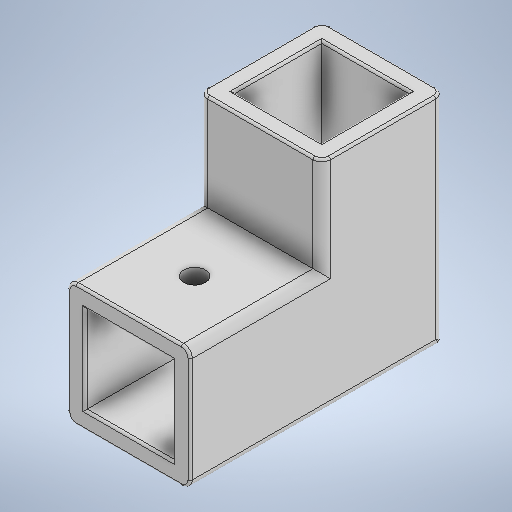
# Autodesk Inventor part: fixed_joint
Saved by Autodesk Inventor 2025 (Build 290162000, 162)
## iProperties
Created: 2024-07-12
Part Number: fixed_joint
Material: Generic
Document SubType Name: Modeling
Designer: hifzhil
Density: 1 g/cm^3
Appearance: Default
Author: hifzhil
Autodesk Inventor part; units mm, degrees
sketch "Sketch1" plane through (0, 0, 0) normal (0, 0, 1) x (1, 0, 0)
  line L0 (-11.6216, -5.5135) -> (8.3784, -5.5135)
  line L1 (8.3784, -5.5135) -> (8.3784, -25.5135)
  line L2 (8.3784, -25.5135) -> (-11.6216, -25.5135)
  line L3 (-11.6216, -25.5135) -> (-11.6216, -5.5135)
  line L4 (-15.6216, -1.5135) -> (12.3784, -1.5135)
  line L5 (12.3784, -1.5135) -> (12.3784, -29.5135)
  line L6 (12.3784, -29.5135) -> (-15.6216, -29.5135)
  line L7 (-15.6216, -29.5135) -> (-15.6216, -1.5135)
  point P0 (0, 0)
  dimension "d0" = 20
  dimension "d1" = 20
  dimension "d2" = 4
  dimension "d3" = 4
  dimension "d4" = 4
  dimension "d5" = 4
  constraints: 16 end point, 4 parallel, 2 horizontal, 2 perpendicular
  measures "d0" distance of L0.end L1.end
  measures "d1" distance of L0.start L0.end
  measures "d2" distance between parallel lines of L0 L4
  measures "d3" distance between parallel lines of L6 L2
  measures "d4" distance between parallel lines of L7 L3
  measures "d5" distance between parallel lines of L5 L1
extrude "Extrusion1" add sketch "Sketch1" along normal blind 30
ref_plane "Work Plane3" through (-15.6216, -29.5135, 0) normal (0, -1, 0) x (1, 0, 0)
sketch "Sketch2" plane through (-15.6216, -29.5135, 0) normal (0, -1, 0) x (1, 0, 0)
  line L0 (0, 0) -> (28, 0)
  line L1 (28, 0) -> (28, -28)
  line L2 (28, -28) -> (0, -28)
  line L3 (0, -28) -> (0, 0)
  line L4 (24, -24) -> (4, -24)
  line L5 (4, -24) -> (4, -4)
  line L6 (4, -4) -> (24, -4)
  line L7 (24, -4) -> (24, -24)
  point P0 (15.6216, 0)
  point P1 (0, -14)
  dimension "d10" = 28
  dimension "d11" = 28
  dimension "d12" = 4
  dimension "d13" = 4
  dimension "d14" = 4
  dimension "d15" = 4
  constraints: 16 end point, 4 parallel, 2 horizontal, 2 perpendicular, 1 midpoint
  measures "d10" distance of L0.end L1.end
  measures "d11" distance of L1.end L2.end
  measures "d12" distance between parallel lines of L1 L7
  measures "d13" distance from line of point (0, -14) L5
  measures "d14" distance between parallel lines of L4 L2
  measures "d15" distance between parallel lines of L0 L6
extrude "Extrusion2" add sketch "Sketch2" against normal blind 50
ref_plane "Work Plane4" through (12.3784, -29.5135, -28) normal (0, 0, -1) x (-1, 0, 0)
sketch "Sketch3" plane through (12.3784, -29.5135, -28) normal (0, 0, -1) x (-1, 0, 0)
  circle A0 centre (14, 35) radius 2.5
  circle A1 centre (14, 15) radius 2.5
  line L0 (28, 0) -> (28, 50) projected
  line L1 (28, 0) -> (0, 0) projected
  point P0 (12.3784, 29.5135)
  dimension "d19" = 14
  dimension "d20" = 14
  dimension "d21" = 20
  dimension "d22" = 15
  dimension "d23" = 5
  dimension "d24" = 5
  constraints: 2 centre point
  measures "d19" distance from line of L0 A1.centre
  measures "d20" distance from line of L0 A0.centre
  measures "d21" distance of A0.centre A1.centre
  measures "d22" distance from line of L1 A1.centre
  measures "d23" diameter of A1
  measures "d24" diameter of A0
ref_plane "Work Plane5" through (-15.6216, -1.5135, 30) normal (0, 1, 0) x (1, 0, 0)
sketch "Sketch4" plane through (-15.6216, -1.5135, 30) normal (0, 1, 0) x (1, 0, 0)
  circle A0 centre (14, 15) radius 2.5
  line L0 (28, 30) -> (28, 0) projected
  line L1 (28, 0) -> (0, 0) projected
  point P0 (15.6216, 30)
  dimension "d26" = 5
  dimension "d27" = 14
  dimension "d28" = 15
  constraints: 1 centre point
  measures "d26" diameter of A0
  measures "d27" distance from line of L0 A0.centre
  measures "d28" distance from line of L1 A0.centre
ref_plane "Work Plane6" through (-15.6216, -29.5135, 30) normal (0, -1, 0) x (1, 0, 0)
sketch "Sketch5" plane through (-15.6216, -29.5135, 30) normal (0, -1, 0) x (1, 0, 0)
  circle A0 centre (14, -15) radius 2.5
  line L0 (0, -30) -> (0, 0) projected
  line L1 (24, 0) -> (4, 0) projected
  point P0 (15.6216, -30)
  dimension "d30" = 5
  dimension "d31" = 14
  dimension "d32" = 15
  constraints: 1 centre point
  measures "d30" diameter of A0
  measures "d31" distance from line of L0 A0.centre
  measures "d32" distance from line of L1 A0.centre
extrude "Extrusion3" cut sketch "Sketch4" against normal blind 4
extrude "Extrusion4" cut sketch "Sketch5" against normal blind 4
extrude "Extrusion5" cut sketch "Sketch3" against normal blind 4
fillet "Fillet1" radius 2 8 edges at (12.3784, -1.5135, 15) (12.3784, 9.4865, 0) (12.3784, -29.5135, 1) (12.3784, -4.5135, -28) (-15.6216, 9.4865, 0) (-15.6216, -1.5135, 15) (-15.6216, -4.5135, -28) (-15.6216, -29.5135, 1)
fillet "Fillet2" radius 0.5 31 edges at (-1.6216, -29.5135, -24) (8.3784, -29.5135, -14) (-11.6216, -29.5135, -14) (-1.6216, -29.5135, -4) (11.7926, -28.9277, -27.4142) (-15.0358, -28.9277, -27.4142) (-1.6216, -29.5135, -28) (-1.6216, 20.4865, -24) (-11.6216, 20.4865, -14) (8.3784, 20.4865, -14) (-1.6216, 20.4865, -4) (-15.0358, 20.4865, -27.4142) (-15.6216, 20.4865, -14) (-15.0358, 20.4865, -0.5858) (-1.6216, 20.4865, 0) (11.7926, 20.4865, -0.5858) (12.3784, 20.4865, -14) (11.7926, 20.4865, -27.4142) (-1.6216, 20.4865, -28) (-1.6216, -25.5135, 30) (8.3784, -15.5135, 30) (-1.6216, -5.5135, 30) (-11.6216, -15.5135, 30) (11.7926, -28.9277, 30) (12.3784, -15.5135, 30) (11.7926, -2.0993, 30) (-1.6216, -1.5135, 30) (-15.0358, -2.0993, 30) (-15.6216, -15.5135, 30) (-15.0358, -28.9277, 30) (-1.6216, -29.5135, 30)
ref_plane "Work Plane7" through (-13.6216, -29.5135, 29.5) normal (0, -1, 0) x (1, 0, 0)
sketch "Sketch6" plane through (-13.6216, -29.5135, 29.5) normal (0, -1, 0) x (1, 0, 0)
  line L0 (23.2157, -54.9948) -> (0.8161, -54.9948)
  line L1 (0.8161, -54.9948) -> (0.8161, -31.6008)
  line L2 (0.8161, -31.6008) -> (23.2157, -31.6008)
  line L3 (23.2157, -31.6008) -> (23.2157, -54.9948)
  point P0 (13.6216, -29.5)
  constraints: 8 end point, 2 parallel, 1 horizontal, 1 perpendicular
extrude "Extrusion6" add sketch "Sketch6" against normal blind 4
body "Solid1"
